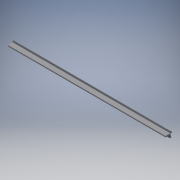
# Autodesk Inventor part: junta controler
Saved by Autodesk Inventor 2016 (Build 200138000, 138)
## iProperties
Created: 2017-06-07
Part Number: junta controler
Material: Generic
Document SubType Name: Modeling
Designer: fabio-note
Density: 1 g/cm^3
Appearance: Default
Author: fabio-note
Autodesk Inventor part; units mm, degrees
ref_plane "YZ Plane" through (0, 0, 0) normal (1, 0, 0) x (0, 1, 0)
ref_plane "XZ Plane" through (0, 0, 0) normal (0, 1, 0) x (-1, 0, 0)
ref_plane "XY Plane" through (0, 0, 0) normal (0, 0, 1) x (1, 0, 0)
sketch "Sketch1" plane through (0, 0, 0) normal (1, 0, 0) x (0, 1, 0)
  line L0 (5, -15.415) -> (5, -19.415)
  line L1 (5, -19.415) -> (-5, -19.415)
  line L2 (5, -20.415) -> (8.7898, -19.1353)
  line L3 (5, -20.415) -> (7.3565, -27.3935)
  line L4 (7.3565, -27.3935) -> (4.6727, -28.2998)
  line L5 (4.6727, -28.2998) -> (2.4715, -21.7812)
  line L6 (2.4715, -21.7812) -> (-5, -21.7812)
  line L7 (-5, -21.7812) -> (-5, -19.415)
  arc A0 (8.7898, -19.1353) -> (5, -15.415) centre (1.7532, -22.5129) ccw
  point P0 (0, 0)
  point P1 (0, -20.415)
  dimension "d0" = 4
  dimension "d4" = 4
  constraints: 16 end point, 3 perpendicular, 2 point on circle, 2 vertical, 1 centre point, 1 horizontal, 1 vertical alignment
  measures "d0" distance of L0.start L0.end
  measures "d4" distance of L2.end L2.start
extrude "Extrusion1" add sketch "Sketch1" along normal blind 330
body "Solid1"
